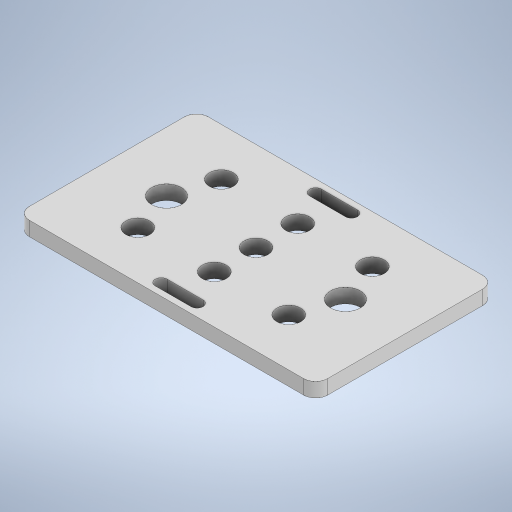
# Autodesk Inventor part: Cart
Saved by Autodesk Inventor 2024.3 (Build 283343000, 343)
## iProperties
Created: 2024-12-08
Part Number: Cart
Material: Generic
Document SubType Name: Modeling
Designer: Nada
Density: 1 g/cm^3
Appearance: Default
Author: Nada
Autodesk Inventor part; units mm, degrees
ref_plane "YZ Plane" through (0, 0, 0) normal (1, 0, 0) x (0, 1, 0)
ref_plane "XZ Plane" through (0, 0, 0) normal (0, 1, 0) x (-1, 0, 0)
ref_plane "XY Plane" through (0, 0, 0) normal (0, 0, 1) x (1, 0, 0)
sketch "Sketch1" plane through (0, 0, 0) normal (0, 1, 0) x (-1, 0, 0)
  line L0 (0, -2) -> (0, -28)
  line L1 (2, -30) -> (48, -30)
  line L2 (50, -28) -> (50, -2)
  line L3 (48, 0) -> (2, 0)
  arc A0 (50, -2) -> (48, 0) centre (48, -2) ccw
  arc A1 (48, -30) -> (50, -28) centre (48, -28) ccw
  arc A2 (0, -28) -> (2, -30) centre (2, -28) ccw
  arc A3 (2, 0) -> (0, -2) centre (2, -2) ccw
  point P0 (0, 0)
  point P1 (0, -30)
  point P2 (50, -30)
  point P3 (50, 0)
  dimension "d0" = 30
  dimension "d1" = 50
  dimension "d4" = 2
  constraints: 8 end point, 8 point on circle, 8 point on line, 8 tangent, 4 centre point, 3 equal radius, 3 perpendicular, 1 vertical
  measures "d0" distance of point (0, 0) point (0, -30)
  measures "d1" distance of point (0, -30) point (50, -30)
  measures "d4" radius of A0
extrude "Extrusion1" add sketch "Sketch1" along normal blind 2.4
sketch "Sketch2" plane through (0, 2.4, 0) normal (0, 1, 0) x (1, 0, 0)
  line L0 (0, 2) -> (0, 28) projected
  line L1 (-50, 28) -> (-50, 2) projected
  line L2 (-50, 17.5) -> (-50, 12.5)
  line L3 (-50, 15) -> (-25, 15)
  line L4 (-25, 15) -> (-40, 15)
  line L5 (-40, 15) -> (-25, 15)
  line L6 (-25, 15) -> (-10, 15)
  circle A0 centre (-40, 15) radius 2.5
  circle A1 centre (-10, 15) radius 2.5
  dimension "d22" = 5
  dimension "d62" = 25
  dimension "d63" = 15
  dimension "d64" = 15
  dimension "d65" = 5
  dimension "d66" = 5
  constraints: 10 end point, 3 point on line, 2 centre point, 2 coincident, 2 horizontal, 1 collinear, 1 midpoint
  measures "d22" distance of L2.start L2.end
  measures "d62" distance of L3.start L3.end
  measures "d63" distance of L3.end L4.end
  measures "d64" distance of L3.end L6.end
  measures "d65" diameter of A0
  measures "d66" diameter of A1
extrude "Extrusion2" cut sketch "Sketch2" against normal blind 2.4
sketch "Sketch3" plane through (0, 2.4, 0) normal (0, 1, 0) x (1, 0, 0)
  line L0 (0, 0) -> (-25, 0)
  line L1 (-48, 0) -> (-2, 0) projected
  line L2 (-25, 0) -> (-25, 29.9791)
  line L3 (-28, 27.9998) -> (-22, 27.9998) construction
  line L4 (-28, 26.9998) -> (-22, 26.9998)
  line L5 (-22, 28.9998) -> (-28, 28.9998)
  arc A0 (-28, 28.9998) -> (-28, 26.9998) centre (-28, 27.9998) ccw
  arc A1 (-22, 26.9998) -> (-22, 28.9998) centre (-22, 27.9998) ccw
  line L6 (-2, 30) -> (-48, 30) projected
  line L7 (-27.8848, 2) -> (-21.8848, 2) construction
  line L8 (-27.8848, 1) -> (-21.8848, 1)
  line L9 (-21.8848, 3) -> (-27.8848, 3)
  arc A2 (-27.8848, 3) -> (-27.8848, 1) centre (-27.8848, 2) ccw
  arc A3 (-21.8848, 1) -> (-21.8848, 3) centre (-21.8848, 2) ccw
  point P0 (-25, 27.9998)
  point P1 (-24.8848, 2)
  dimension "d28" = 25
  dimension "d29" = 3
  dimension "d30" = 2
  dimension "d31" = 2.0002
  dimension "d32" = 3
  dimension "d33" = 2
  dimension "d34" = 2
  constraints: 20 end point, 8 point on circle, 8 tangent, 4 centre point, 3 midpoint, 3 perpendicular, 2 parallel, 1 point on line
  measures "d28" distance of L0.start L0.end
  measures "d29" distance of point (-25, 28) L3.end
  measures "d30" diameter of A1
  measures "d31" distance from line of L6 point (-25, 28)
  measures "d32" distance of point (-24.885, 2) L7.end
  measures "d33" diameter of A3
  measures "d34" distance between parallel lines of L1 L7
extrude "Extrusion3" cut sketch "Sketch3" along normal mid plane 66
sketch "Sketch5" plane through (0, 2.4, 0) normal (0, 1, 0) x (1, 0, 0)
  line L0 (0, 2) -> (0, 28) projected
  line L1 (0, 15) -> (-25, 15)
  line L2 (-25, 15) -> (-25, 22)
  circle A0 centre (-25, 22) radius 2
  line L3 (-25, 15) -> (-25, 8)
  circle A1 centre (-25, 8) radius 2
  point P0 (0, 0)
  dimension "d43" = 25
  dimension "d44" = 7
  dimension "d45" = 4
  dimension "d46" = 7
  dimension "d47" = 4
  constraints: 6 end point, 2 centre point, 2 coincident, 1 horizontal, 1 midpoint, 1 perpendicular, 1 vertical
  measures "d43" distance of L1.start L1.end
  measures "d44" distance of L1.end L2.end
  measures "d45" diameter of A0
  measures "d46" distance of L1.end L3.end
  measures "d47" diameter of A1
extrude "Extrusion5" cut sketch "Sketch5" against normal blind 66
sketch "Sketch6" plane through (0, 2.4, 0) normal (0, 1, 0) x (1, 0, 0)
  line L0 (0, 2) -> (0, 28) projected
  line L1 (0, 15) -> (-12.5, 15)
  line L2 (-12.5, 15) -> (-12.5, 22)
  line L3 (-12.5, 22) -> (-12.5, 8)
  circle A0 centre (-12.5, 22) radius 2
  circle A1 centre (-12.5, 8) radius 2
  line L4 (-50.3101, 15) -> (-37.8101, 15)
  line L5 (-37.8101, 15) -> (-37.8101, 22)
  line L6 (-37.8101, 22) -> (-37.8101, 8)
  circle A2 centre (-37.8101, 22) radius 2
  circle A3 centre (-37.8101, 8) radius 2
  point P0 (0, 0)
  dimension "d50" = 12.5
  dimension "d51" = 7
  dimension "d52" = 14
  dimension "d53" = 4
  dimension "d54" = 4
  dimension "d55" = 12.5
  dimension "d56" = 7
  dimension "d57" = 14
  dimension "d58" = 4
  dimension "d59" = 4
  constraints: 12 end point, 4 centre point, 4 coincident, 2 horizontal, 2 perpendicular, 2 point on line, 1 midpoint
  measures "d50" distance of L1.start L1.end
  measures "d51" distance of L1.end L2.end
  measures "d52" distance of L2.end L3.end
  measures "d53" diameter of A0
  measures "d54" diameter of A1
  measures "d55" distance of L4.start L4.end
  measures "d56" distance of L4.end L5.end
  measures "d57" distance of L5.end L6.end
  measures "d58" diameter of A2
  measures "d59" diameter of A3
extrude "Extrusion6" cut sketch "Sketch6" against normal blind 66
sketch "Sketch7" plane through (0, 2.4, 0) normal (0, 1, 0) x (1, 0, 0)
  line L0 (-48, 0) -> (-2, 0) projected
  line L1 (-48, 0) -> (-48, 15)
  line L2 (-48, 15) -> (-25, 15)
  circle A0 centre (-25, 15) radius 2
  point P0 (0, 0)
  dimension "d67" = 15
  dimension "d68" = 4
  constraints: 4 end point, 1 centre point, 1 coincident, 1 perpendicular, 1 vertical
  measures "d67" distance of L0.start L1.end
  measures "d68" diameter of A0
extrude "Extrusion7" cut sketch "Sketch7" against normal through all
body "Solid1"
